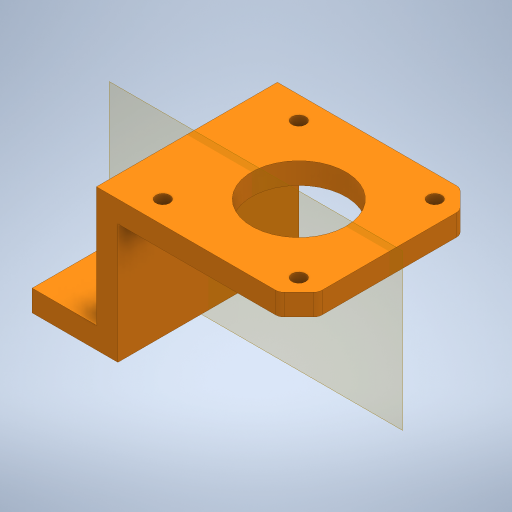
# Autodesk Inventor part: StepperZHolder
Saved by Autodesk Inventor 2023 (Build 270158000, 158)
## iProperties
Created: 2022-09-02
Part Number: StepperZHolder
Material: Generic
Document SubType Name: Modeling
Designer: Nathann
Density: 1 g/cm^3
Appearance: Orange
Author: Nathann
Autodesk Inventor part; units mm, degrees
ref_plane "YZ Plane" through (0, 0, 0) normal (1, 0, 0) x (0, 1, 0)
ref_plane "XZ Plane" through (0, 0, 0) normal (0, 1, 0) x (-1, 0, 0)
ref_plane "XY Plane" through (0, 0, 0) normal (0, 0, 1) x (1, 0, 0)
sketch "Sketch1" plane through (0, 0, 0) normal (0, 0, 1) x (1, 0, 0)
  arc A0 (-20.5392, 17.1146) -> (-21.125, 15.7004) centre (-19.125, 15.7004) ccw projected
  line L0 (-21.125, -15.7004) -> (-21.125, 15.7004) projected
  arc A1 (-21.125, -15.7004) -> (-20.5392, -17.1146) centre (-19.125, -15.7004) ccw projected
  line L1 (-20.5392, -17.1146) -> (-17.1146, -20.5392) projected
  arc A2 (-17.1146, -20.5392) -> (-15.7004, -21.125) centre (-15.7004, -19.125) ccw projected
  line L2 (15.7004, -21.125) -> (-15.7004, -21.125) projected
  arc A3 (15.7004, -21.125) -> (17.1146, -20.5392) centre (15.7004, -19.125) ccw projected
  line L3 (20.5392, -17.1146) -> (17.1146, -20.5392) projected
  arc A4 (20.5392, -17.1146) -> (21.125, -15.7004) centre (19.125, -15.7004) ccw projected
  line L4 (21.125, 15.7004) -> (21.125, -15.7004) projected
  arc A5 (21.125, 15.7004) -> (20.5392, 17.1146) centre (19.125, 15.7004) ccw projected
  line L5 (20.5392, 17.1146) -> (17.1146, 20.5392) projected
  arc A6 (17.1146, 20.5392) -> (15.7004, 21.125) centre (15.7004, 19.125) ccw projected
  line L6 (-15.7004, 21.125) -> (15.7004, 21.125) projected
  arc A7 (-15.7004, 21.125) -> (-17.1146, 20.5392) centre (-15.7004, 19.125) ccw projected
  line L7 (-20.5392, 17.1146) -> (-17.1146, 20.5392) projected
  circle A8 centre (0, 0) radius 16 projected
  circle A9 centre (-15.875, -15.875) radius 1.625 projected
  circle A10 centre (15.875, 15.875) radius 1.625 projected
  circle A11 centre (-15.875, 15.875) radius 1.625 projected
  circle A12 centre (15.875, -15.875) radius 1.625 projected
  circle A13 centre (0, 0) radius 11 projected
  point P0 (0, 0)
extrude "Extrusion1" add sketch "Sketch1" along normal blind 5 contours L7 A7 L6 A6 L5 A5 L4 A4 L3 A3 L2 A2 L1 A1 L0 A0 | A8
sketch "Sketch2" plane through (-21.125, -15.7004, 0) normal (-1, 0, 0) x (0, 0, 1)
  line L0 (0, -5.4246) -> (5, -5.4246) projected
  line L1 (5, -5.4246) -> (-28, -5.4246)
  line L2 (-28, -5.4246) -> (-28, 36.8254)
  line L3 (-28, 36.8254) -> (5, 36.8254)
  line L4 (5, 36.8254) -> (5, -5.4246)
  point P0 (0, 15.7004)
  dimension "d6" = 33
  constraints: 8 end point, 2 parallel, 1 horizontal, 1 perpendicular
  measures "d6" distance of L2.end L3.end
extrude "Extrusion2" add sketch "Sketch2" along normal blind 5
sketch "Sketch3" plane through (0, 0, 5) normal (0, 0, 1) x (1, 0, 0)
  line L0 (-21.125, -15.7004) -> (-21.125, -21.125) projected
  arc A0 (-21.125, -15.7004) -> (-20.5392, -17.1146) centre (-19.125, -15.7004) ccw projected
  arc A1 (-17.1146, -20.5392) -> (-15.7004, -21.125) centre (-15.7004, -19.125) ccw projected
  line L1 (-20.5392, -17.1146) -> (-17.1146, -20.5392) projected
  line L2 (-21.125, -21.125) -> (-15.7004, -21.125)
  line L3 (-21.125, 21.125) -> (-21.125, 15.7004) projected
  arc A2 (-15.7004, 21.125) -> (-17.1146, 20.5392) centre (-15.7004, 19.125) ccw projected
  line L4 (-21.125, 21.125) -> (-15.7004, 21.125)
  line L5 (-17.1146, 20.5392) -> (-20.5392, 17.1146) projected
  arc A3 (-20.5392, 17.1146) -> (-21.125, 15.7004) centre (-19.125, 15.7004) ccw projected
  point P0 (0, 0)
  constraints: 4 end point, 2 horizontal, 1 tangent
extrude "Extrusion3" add sketch "Sketch3" against normal blind 5
sketch "Sketch4" plane through (-26.125, -15.7004, 0) normal (-1, 0, 0) x (0, 0, 1)
  line L0 (0, -5.4246) -> (-28, -5.4246) projected
  line L1 (5, 36.8254) -> (-28, 36.8254) projected
  line L2 (-28, -5.4246) -> (-23, -5.4246)
  line L3 (-23, -5.4246) -> (-23, 36.8254)
  line L4 (-23, 36.8254) -> (-28, 36.8254)
  line L5 (-28, 36.8254) -> (-28, -5.4246)
  point P0 (0, 15.7004)
  dimension "d7" = 5
  constraints: 8 end point, 2 parallel, 1 horizontal, 1 perpendicular, 1 point on line
  measures "d7" distance between parallel lines of L5 L3
extrude "Extrusion4" add sketch "Sketch4" along normal blind 15
sketch "Sketch5" plane through (-26.125, -21.125, -23) normal (0, 0, 1) x (1, 0, 0)
  circle A0 centre (-5, 32.25) radius 2.25
  circle A1 centre (-5, 10) radius 2.25
  line L0 (0, 42.25) -> (-15, 42.25) projected
  line L1 (-15, 0) -> (-15, 42.25) projected
  line L2 (0, 0) -> (-15, 0) projected
  point P0 (26.125, 21.125)
  dimension "d10" = 10
  dimension "d11" = 10
  dimension "d12" = 10
  dimension "d13" = 10
  dimension "d14" = 4.5
  dimension "d15" = 4.5
  constraints: 2 centre point
  measures "d10" distance from line of L0 A0.centre
  measures "d11" distance from line of L1 A0.centre
  measures "d12" distance from line of L1 A1.centre
  measures "d13" distance from line of L2 A1.centre
  measures "d14" diameter of A0
  measures "d15" diameter of A1
extrude "Extrusion5" cut sketch "Sketch5" along normal through all both and the other way through all
ref_plane "Work Plane1" through (15.7004, 0, 0) normal (0, -1, 0) x (1, 0, 0)
sketch "Sketch6" plane through (15.7004, 0, 0) normal (0, -1, 0) x (1, 0, 0)
  line L0 (-41.8254, -23) -> (-56.8254, -23) projected
  line L1 (0, 5) -> (-41.8254, 5) projected
  line L2 (-56.8254, -23) -> (-41.8254, 5)
  line L3 (-41.8254, 5) -> (-41.8254, -23)
  line L4 (-41.8254, -23) -> (-56.8254, -23)
  point P0 (-15.7004, 0)
  constraints: 6 end point, 2 perpendicular
extrude "Extrusion6" add sketch "Sketch6" along normal mid plane 10
equation "\"d15\" = d14"
body "Solid1"
